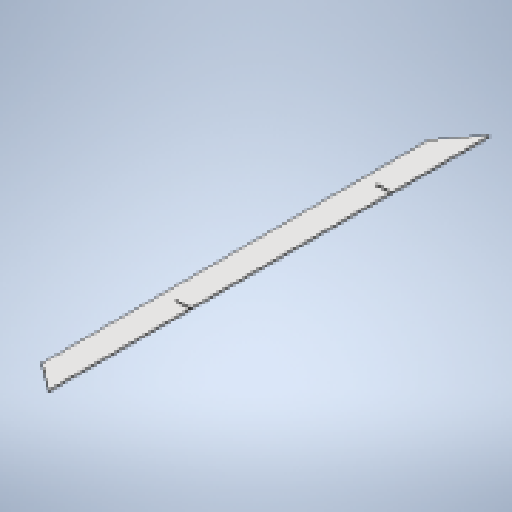
# Autodesk Inventor part: MSC 603 stringer cone exit back
Saved by Autodesk Inventor 2025 (Build 290162010, 162A)
## iProperties
Created: 2024-08-26
Part Number: MSC 603 stringer cone exit back
Material: Stainless Steel
Document SubType Name: Sheet Metal
Designer: pokla
Density: 8 g/cm^3
Sheet Metal Rule: AISI304 3mm Die 32
Appearance: Default
Stock Number: МОО 603 стрингер конус выход корма
Mass: 929.186 g
Surface Area: 828.252 cm^2
Volume: 116.148 cm^3
Flat Pattern Width: 85.7582 cm
Flat Pattern Length: 5 cm
Flat Pattern Area: 428.791 cm^2
Sheet Metal Width: 857,582 mm
Sheet Metal Length: 50,000 mm
Sheet Metal Area: 42879,111 mm^2
Author: pokla
Autodesk Inventor part; units mm, degrees
ref_plane "YZ Plane" through (0, 0, 0) normal (1, 0, 0) x (0, 1, 0)
ref_plane "XZ Plane" through (0, 0, 0) normal (0, 1, 0) x (-1, 0, 0)
ref_plane "XY Plane" through (0, 0, 0) normal (0, 0, 1) x (1, 0, 0)
sketch "Sketch1" plane through (0, 0, 0) normal (0, 0, 1) x (1, 0, 0)
  line L0 (-25, 0) -> (25, 0)
  line L1 (25, 0) -> (25, -860)
  line L2 (25, -860) -> (-25, -860)
  line L3 (-25, -860) -> (-25, 0)
  line L4 (25, 0) -> (-25, -68.0668)
  point P0 (0, 0)
  point P1 (0, 0)
  point P2 (25, -1153.2713)
  dimension "d0" = 50
  dimension "d1" = 860
  dimension "d6" = 53.7
  measures "d0" distance of L0.start L0.end
  measures "d1" distance of L2.end L0.start
  measures "d6" angle of L0 L4
extrude "Plate1" add sketch "Sketch1" along normal mid plane 3 contours L1 L2 L3 L4
chamfer "Corner Chamfer2" distance 3 angle 45 1 edges at (25, 0, 0)
fillet "Corner Round1" radius 6 1 edges at (-25, -68.0668, 0)
sketch "Sketch2" plane through (0, 0, 1.5) normal (0, 0, 1) x (1, 0, 0)
  line L0 (25, -186.5) -> (-1, -186.5)
  line L1 (-1, -186.5) -> (-1, -189.5)
  line L2 (-1, -189.5) -> (25, -189.5)
  line L3 (25, -189.5) -> (25, -186.5)
  line L4 (25, -3) -> (25, -860) projected
  point P0 (0, 0)
  point P1 (25, -188)
  point P2 (25, -827)
  dimension "d15" = 188
  dimension "d16" = 26
  dimension "d17" = 3
  constraints: 8 end point, 2 parallel, 1 horizontal, 1 midpoint, 1 perpendicular, 1 point on line
  measures "d15" vertical distance of point (0, 0) point (25, -188)
  measures "d16" distance of L1.end L2.end
  measures "d17" distance of L0.end L1.end
extrude "Extrusion1" cut sketch "Sketch2" against normal through all
pattern_linear "Rectangular Pattern1" count 3 spacing 323 along (0, -1, 0) of "Extrusion1"
fillet "Corner Round3" radius 6 1 edges at (-25, -860, 0)
equation "\"d6\" = d5"
equation "\"d2\" = Thickness"
equation "\"BendReliefWidth\" = Thickness"
equation "\"BendReliefDepth\" = 0.5 * Thickness"
equation "\"CornerReliefSize\" = 4 * Thickness"
equation "\"MinimumRemnant\" = 2 * Thickness"
equation "\"TransitionRadius\" = BendRadius"
equation "\"JacobiRadiusSize\" = BendRadius"
equation "\"GapSize\" = Thickness"
equation "\"d5\" = 53.7deg"
equation "\"Thickness\" = 3"
equation "\"BendRadius\" = 5"
body "Solid1"
